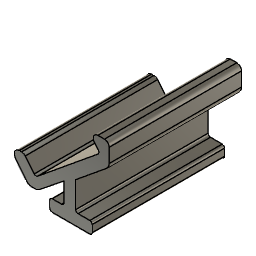
sostegno_DCDC (Autodesk Fusion 360 design; units mm, degrees)
part number: 2025-06-22-10-27-07-458
Autodesk Fusion 360 part; units mm, degrees
sketch "Schizzo1" plane through (0, 0, 0) normal (0, 0, 1) x (1, 0, 0)
  line L0 (0, 0) -> (35.2, 0)
  line L1 (35.2, 0) -> (35.2, 56.2)
  line L2 (35.2, 56.2) -> (0, 56.2)
  line L3 (0, 56.2) -> (0, 0)
  dimension "d1" = 35.2
  dimension "d2" = 56.2
  constraint horizontal L0
  constraint vertical L1
  constraint horizontal L2
  constraint vertical L3
  constraint coincident L0.start L3.end
  measures "d1" distance of L0.start L0.end
  measures "d2" distance of L0.start L2.end
extrude "Estrusione1" add sketch "Schizzo1" along normal blind 40
sketch "Schizzo2" plane through (0, 56.2, 0) normal (0, 1, 0) x (-1, 0, 0)
  line L0 (-35.2, 0) -> (0, 0)
  line L1 (0, 0) -> (0, 40)
  line L2 (0, 40) -> (-35.2, 40)
  line L3 (-35.2, 40) -> (-35.2, 0)
  line L4 (-35.2, 40) -> (-31.2, 40)
  line L5 (-31.2, 40) -> (-3.9522, 17.7156)
  line L6 (-3.9522, 17.7156) -> (0, 17.7156)
  dimension "d5" = 4
  dimension "d6" = 35.2
  constraint coincident L2.end L3.start
  constraint perpendicular L3 L4
  constraint coincident L1 L6.end
  constraint perpendicular L1 L6
  measures "d5" distance of L2.end L4.end
  measures "d6" distance of L4.end L5.end
extrude "Estrusione2" cut sketch "Schizzo2" against normal blind 70 contours L1 L2 L5 L6
extrude "Estrusione3" cut 1 faces at (22.1174, 37.4667, 32.5719) along direction (0.63308, 0, -0.774086) blind 5
extrude "Estrusione4" add 1 faces at (35.2, 18.7333, 13.3333) along direction (1, 0, 0) blind 5
fillet "Raccordo1" radius 2 4 edges at (3.9522, 28.1, 17.7156) (0, 28.1, 17.7156) (31.2, 28.1, 40) (40.2, 28.1, 40)
extrude "Estrusione5" cut 1 faces at (25.2828, 37.4667, 28.7014) along direction (0.63308, 0, -0.774086) blind 3
fillet "Raccordo2" radius 1 1 edges at (36.2646, 28.1, 33.8073)
fillet "Raccordo3" radius 1 1 edges at (9.0168, 28.1, 11.5229)
sketch "Schizzo7" plane through (0, 56.2, 0) normal (0, 1, 0) x (-1, 0, 0)
  line L0 (-4.5523, 16.9817) -> (-8.3837, 12.297)
  arc A0 (-9.7909, 12.156) -> (-8.3837, 12.297) centre (-9.1578, 12.9301) ccw
  line L1 (-9.7909, 12.156) -> (-35.4906, 33.1742)
  arc A1 (-35.6316, 34.5814) -> (-35.4906, 33.1742) centre (-34.8575, 33.9483) ccw
  line L2 (-35.6316, 34.5814) -> (-33.8712, 36.7338)
  arc A2 (-33.8712, 36.7338) -> (-35.4194, 40) centre (-35.4194, 38) ccw
  line L3 (-35.4194, 40) -> (-38.2, 40)
  arc A3 (-38.2, 40) -> (-40.2, 38) centre (-38.2, 38) ccw
  line L4 (-40.2, 38) -> (-40.2, 0)
  line L5 (-40.2, 0) -> (0, 0)
  line L6 (0, 0) -> (0, 15.7156)
  arc A4 (0, 15.7156) -> (-2, 17.7156) centre (-2, 15.7156) ccw
  line L7 (-2, 17.7156) -> (-3.0042, 17.7156)
  arc A5 (-3.0042, 17.7156) -> (-4.5523, 16.9817) centre (-3.0042, 15.7156) ccw
  line L8 (-40.2, 30.6261) -> (-26, 19)
  line L9 (-26, 19) -> (-26, 7)
  line L10 (-26, 7) -> (-33, 7)
  line L11 (-33, 7) -> (-33, 2)
  line L12 (-33, 2) -> (-15, 2)
  line L13 (-15, 2) -> (-15, 7)
  line L14 (-15, 7) -> (-21, 7)
  line L15 (-21, 7) -> (-21, 16)
  line L16 (-21, 16) -> (-11, 8)
  line L17 (-11, 8) -> (-9.75, 7)
  line L18 (-9.75, 7) -> (-6, 7)
  line L19 (-6, 7) -> (0, 14.5)
  constraint coincident L4 L8.start
  constraint parallel L4 L9
  constraint perpendicular L9 L10
  constraint perpendicular L10 L11
  constraint perpendicular L9 L12
  constraint perpendicular L10 L13
  constraint perpendicular L9 L14
  constraint perpendicular L10 L15
  constraint parallel L16 L17
  constraint perpendicular L6 L18
  constraint coincident L6 L19.end
  constraint perpendicular L16 L19
extrude "Estrusione6" cut sketch "Schizzo7" against normal blind 95 contours L4 L5 L6 L8 L9 L10 L11 L12 L13 L14 L15 L16 L17 L18 L19
fillet "Raccordo4" radius 3 4 edges at (0, 28.1, 14.5) (6, 28.1, 7) (9.75, 28.1, 7) (40.2, 28.1, 30.6261)
fillet "Raccordo5" radius 1 6 edges at (26, 28.1, 7) (33, 28.1, 7) (21, 28.1, 7) (15, 28.1, 7) (15, 28.1, 2) (33, 28.1, 2)
sketch "Schizzo3" plane through (0, 56.2, 0) normal (0, 1, 0) x (-1, 0, 0)
  line L0 (-4.5523, 16.9817) -> (-8.3837, 12.297)
  arc A0 (-9.7909, 12.156) -> (-8.3837, 12.297) centre (-9.1578, 12.9301) ccw
  line L1 (-9.7909, 12.156) -> (-35.4906, 33.1742)
  arc A1 (-35.6316, 34.5814) -> (-35.4906, 33.1742) centre (-34.8575, 33.9483) ccw
  line L2 (-35.6316, 34.5814) -> (-33.8712, 36.7338)
  arc A2 (-33.8712, 36.7338) -> (-35.4194, 40) centre (-35.4194, 38) ccw
  line L3 (-35.4194, 40) -> (-38.2, 40)
  arc A3 (-38.2, 40) -> (-40.2, 38) centre (-38.2, 38) ccw
  line L4 (-40.2, 38) -> (-40.2, 0)
  line L5 (-40.2, 0) -> (0, 0)
  line L6 (0, 0) -> (0, 15.7156)
  arc A4 (0, 15.7156) -> (-2, 17.7156) centre (-2, 15.7156) ccw
  line L7 (-2, 17.7156) -> (-3.0042, 17.7156)
  arc A5 (-3.0042, 17.7156) -> (-4.5523, 16.9817) centre (-3.0042, 15.7156) ccw
  line L8 (-40.2, 29.9744) -> (-24.8148, 16.4613)
  line L9 (-24.8148, 16.4613) -> (-24.8148, 5)
  line L10 (-20.1, 5) -> (-20.1, 14)
  line L11 (-20.1, 14) -> (-8.3458, 5)
  line L12 (-8.3458, 5) -> (0, 5)
  line L13 (-32, 5) -> (-32, 0)
  line L14 (-13, 5) -> (-13, 0)
  constraint coincident L4 L8.start
  constraint perpendicular L5 L9
  constraint perpendicular L5 L10
  constraint coincident L6 L12.end
  constraint perpendicular L6 L12
  constraint coincident L5 L13.end
  constraint perpendicular L5 L13
  constraint coincident L5 L14.end
  constraint perpendicular L5 L14
sketch "Schizzo4" plane through (0, 56.2, 0) normal (0, 1, 0) x (-1, 0, 0)
  line L0 (-24.8139, 4.9985) -> (-32, 4.9985)
  constraint horizontal L0
sketch "Schizzo5" plane through (0, 56.2, 0) normal (0, 1, 0) x (-1, 0, 0)
  line L0 (-13, 5) -> (-20.1, 5)
  constraint horizontal L0
sketch "Schizzo6" plane through (0, 56.2, 0) normal (0, 1, 0) x (-1, 0, 0)
  line L0 (-13, 0) -> (0, 0)
  line L1 (0, 0) -> (0, 5)
  constraint coincident L0.end L1.start
  constraint horizontal L0
  constraint perpendicular L0 L1
